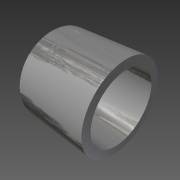
# Autodesk Inventor part: Clutch Sleeve
Saved by Autodesk Inventor 2016 (Build 200138000, 138)
## iProperties
Created: 2012-08-06
Part Number: Clutch Sleeve
Material: Titanium
Document SubType Name: Modeling
Designer: John
Density: 4.51 g/cm^3
Mass: 0.517581 g
Surface Area: 3.26936 cm^2
Volume: 0.114763 cm^3
Appearance: Titanium
Author: John
Autodesk Inventor part; units mm, degrees
ref_plane "YZ Plane" through (0, 0, 0) normal (1, 0, 0) x (0, 1, 0)
ref_plane "XZ Plane" through (0, 0, 0) normal (0, 1, 0) x (-1, 0, 0)
ref_plane "XY Plane" through (0, 0, 0) normal (0, 0, 1) x (1, 0, 0)
sketch "Sketch1" plane through (0, 0, 0) normal (1, 0, 0) x (0, 1, 0)
  circle A0 centre (0, 0) radius 3.9751
  circle A1 centre (0, 0) radius 3.1877
  dimension "d0" = 7.9502
  dimension "d1" = 6.3754
  constraints: 2 centre point, 2 coincident
  measures "d0" diameter of A0
  measures "d1" diameter of A1
extrude "Extrusion1" add sketch "Sketch1" along normal blind 6.477
body "Solid1"
